Autodesk Inventor part; units mm, degrees
(part 2 of 4)
  line L810 (39.2782, -35.709) -> (37.2782, -35.709)
  line L811 (36.2782, -33.9769) -> (37.2782, -32.2449)
  line L812 (42.0103, -32.9769) -> (41.0103, -31.2449)
  line L813 (44.0103, -32.9769) -> (42.0103, -32.9769)
  line L814 (45.0103, -31.2449) -> (44.0103, -32.9769)
  line L815 (41.0103, -31.2449) -> (42.0103, -29.5128)
  line L816 (42.0103, -29.5128) -> (44.0103, -29.5128)
  line L817 (44.0103, -29.5128) -> (45.0103, -31.2449)
  line L818 (46.7423, -35.709) -> (45.7423, -33.9769)
  line L819 (49.7423, -33.9769) -> (48.7423, -35.709)
  line L820 (46.7423, -32.2449) -> (48.7423, -32.2449)
  line L821 (48.7423, -32.2449) -> (49.7423, -33.9769)
  line L822 (48.7423, -35.709) -> (46.7423, -35.709)
  line L823 (45.7423, -33.9769) -> (46.7423, -32.2449)
  line L824 (51.4744, -32.9769) -> (50.4744, -31.2449)
  line L825 (53.4744, -32.9769) -> (51.4744, -32.9769)
  line L826 (54.4744, -31.2449) -> (53.4744, -32.9769)
  line L827 (50.4744, -31.2449) -> (51.4744, -29.5128)
  line L828 (51.4744, -29.5128) -> (53.4744, -29.5128)
  line L829 (53.4744, -29.5128) -> (54.4744, -31.2449)
  line L830 (56.2064, -35.709) -> (55.2064, -33.9769)
  line L831 (59.2064, -33.9769) -> (58.2064, -35.709)
  line L832 (56.2064, -32.2449) -> (58.2064, -32.2449)
  line L833 (58.2064, -32.2449) -> (59.2064, -33.9769)
  line L834 (58.2064, -35.709) -> (56.2064, -35.709)
  line L835 (55.2064, -33.9769) -> (56.2064, -32.2449)
  line L836 (60.9385, -32.9769) -> (59.9385, -31.2449)
  line L837 (62.9385, -32.9769) -> (60.9385, -32.9769)
  line L838 (63.9385, -31.2449) -> (62.9385, -32.9769)
  line L839 (59.9385, -31.2449) -> (60.9385, -29.5128)
  line L840 (60.9385, -29.5128) -> (62.9385, -29.5128)
  line L841 (62.9385, -29.5128) -> (63.9385, -31.2449)
  line L842 (65.6705, -35.709) -> (64.6705, -33.9769)
  line L843 (68.6705, -33.9769) -> (67.6705, -35.709)
  line L844 (65.6705, -32.2449) -> (67.6705, -32.2449)
  line L845 (67.6705, -32.2449) -> (68.6705, -33.9769)
  line L846 (67.6705, -35.709) -> (65.6705, -35.709)
  line L847 (64.6705, -33.9769) -> (65.6705, -32.2449)
  line L848 (70.4026, -32.9769) -> (69.4026, -31.2449)
  line L849 (72.4026, -32.9769) -> (70.4026, -32.9769)
  line L850 (73.4026, -31.2449) -> (72.4026, -32.9769)
  line L851 (69.4026, -31.2449) -> (70.4026, -29.5128)
  line L852 (70.4026, -29.5128) -> (72.4026, -29.5128)
  line L853 (72.4026, -29.5128) -> (73.4026, -31.2449)
  line L854 (75.1346, -35.709) -> (74.1346, -33.9769)
  line L855 (78.1346, -33.9769) -> (77.1346, -35.709)
  line L856 (75.1346, -32.2449) -> (77.1346, -32.2449)
  line L857 (77.1346, -32.2449) -> (78.1346, -33.9769)
  line L858 (77.1346, -35.709) -> (75.1346, -35.709)
  line L859 (74.1346, -33.9769) -> (75.1346, -32.2449)
  line L860 (79.8667, -32.9769) -> (78.8667, -31.2449)
  line L861 (81.8667, -32.9769) -> (79.8667, -32.9769)
  line L862 (82.8667, -31.2449) -> (81.8667, -32.9769)
  line L863 (78.8667, -31.2449) -> (79.8667, -29.5128)
  line L864 (79.8667, -29.5128) -> (81.8667, -29.5128)
  line L865 (81.8667, -29.5128) -> (82.8667, -31.2449)
  line L866 (18.35, -41.1731) -> (17.35, -39.441)
  line L867 (21.35, -39.441) -> (20.35, -41.1731)
  line L868 (18.35, -37.709) -> (20.35, -37.709)
  line L869 (20.35, -37.709) -> (21.35, -39.441)
  line L870 (20.35, -41.1731) -> (18.35, -41.1731)
  line L871 (17.35, -39.441) -> (18.35, -37.709)
  line L872 (23.0821, -38.441) -> (22.0821, -36.709)
  line L873 (25.0821, -38.441) -> (23.0821, -38.441)
  line L874 (26.0821, -36.709) -> (25.0821, -38.441)
  line L875 (22.0821, -36.709) -> (23.0821, -34.9769)
  line L876 (23.0821, -34.9769) -> (25.0821, -34.9769)
  line L877 (25.0821, -34.9769) -> (26.0821, -36.709)
  line L878 (27.8141, -41.1731) -> (26.8141, -39.441)
  line L879 (30.8141, -39.441) -> (29.8141, -41.1731)
  line L880 (27.8141, -37.709) -> (29.8141, -37.709)
  line L881 (29.8141, -37.709) -> (30.8141, -39.441)
  line L882 (29.8141, -41.1731) -> (27.8141, -41.1731)
  line L883 (26.8141, -39.441) -> (27.8141, -37.709)
  line L884 (32.5462, -38.441) -> (31.5462, -36.709)
  line L885 (34.5462, -38.441) -> (32.5462, -38.441)
  line L886 (35.5462, -36.709) -> (34.5462, -38.441)
  line L887 (31.5462, -36.709) -> (32.5462, -34.9769)
  line L888 (32.5462, -34.9769) -> (34.5462, -34.9769)
  line L889 (34.5462, -34.9769) -> (35.5462, -36.709)
  line L890 (37.2782, -41.1731) -> (36.2782, -39.441)
  line L891 (40.2782, -39.441) -> (39.2782, -41.1731)
  line L892 (37.2782, -37.709) -> (39.2782, -37.709)
  line L893 (39.2782, -37.709) -> (40.2782, -39.441)
  line L894 (39.2782, -41.1731) -> (37.2782, -41.1731)
  line L895 (36.2782, -39.441) -> (37.2782, -37.709)
  line L896 (42.0103, -38.441) -> (41.0103, -36.709)
  line L897 (44.0103, -38.441) -> (42.0103, -38.441)
  line L898 (45.0103, -36.709) -> (44.0103, -38.441)
  line L899 (41.0103, -36.709) -> (42.0103, -34.9769)
  line L900 (42.0103, -34.9769) -> (44.0103, -34.9769)
  line L901 (44.0103, -34.9769) -> (45.0103, -36.709)
  line L902 (46.7423, -41.1731) -> (45.7423, -39.441)
  line L903 (49.7423, -39.441) -> (48.7423, -41.1731)
  line L904 (46.7423, -37.709) -> (48.7423, -37.709)
  line L905 (48.7423, -37.709) -> (49.7423, -39.441)
  line L906 (48.7423, -41.1731) -> (46.7423, -41.1731)
  line L907 (45.7423, -39.441) -> (46.7423, -37.709)
  line L908 (51.4744, -38.441) -> (50.4744, -36.709)
  line L909 (53.4744, -38.441) -> (51.4744, -38.441)
  line L910 (54.4744, -36.709) -> (53.4744, -38.441)
  line L911 (50.4744, -36.709) -> (51.4744, -34.9769)
  line L912 (51.4744, -34.9769) -> (53.4744, -34.9769)
  line L913 (53.4744, -34.9769) -> (54.4744, -36.709)
  line L914 (56.2064, -41.1731) -> (55.2064, -39.441)
  line L915 (59.2064, -39.441) -> (58.2064, -41.1731)
  line L916 (56.2064, -37.709) -> (58.2064, -37.709)
  line L917 (58.2064, -37.709) -> (59.2064, -39.441)
  line L918 (58.2064, -41.1731) -> (56.2064, -41.1731)
  line L919 (55.2064, -39.441) -> (56.2064, -37.709)
  line L920 (60.9385, -38.441) -> (59.9385, -36.709)
  line L921 (62.9385, -38.441) -> (60.9385, -38.441)
  line L922 (63.9385, -36.709) -> (62.9385, -38.441)
  line L923 (59.9385, -36.709) -> (60.9385, -34.9769)
  line L924 (60.9385, -34.9769) -> (62.9385, -34.9769)
  line L925 (62.9385, -34.9769) -> (63.9385, -36.709)
  line L926 (65.6705, -41.1731) -> (64.6705, -39.441)
  line L927 (68.6705, -39.441) -> (67.6705, -41.1731)
  line L928 (65.6705, -37.709) -> (67.6705, -37.709)
  line L929 (67.6705, -37.709) -> (68.6705, -39.441)
  line L930 (67.6705, -41.1731) -> (65.6705, -41.1731)
  line L931 (64.6705, -39.441) -> (65.6705, -37.709)
  line L932 (70.4026, -38.441) -> (69.4026, -36.709)
  line L933 (72.4026, -38.441) -> (70.4026, -38.441)
  line L934 (73.4026, -36.709) -> (72.4026, -38.441)
  line L935 (69.4026, -36.709) -> (70.4026, -34.9769)
  line L936 (70.4026, -34.9769) -> (72.4026, -34.9769)
  line L937 (72.4026, -34.9769) -> (73.4026, -36.709)
  line L938 (75.1346, -41.1731) -> (74.1346, -39.441)
  line L939 (78.1346, -39.441) -> (77.1346, -41.1731)
  line L940 (75.1346, -37.709) -> (77.1346, -37.709)
  line L941 (77.1346, -37.709) -> (78.1346, -39.441)
  line L942 (77.1346, -41.1731) -> (75.1346, -41.1731)
  line L943 (74.1346, -39.441) -> (75.1346, -37.709)
  line L944 (79.8667, -38.441) -> (78.8667, -36.709)
  line L945 (81.8667, -38.441) -> (79.8667, -38.441)
  line L946 (82.8667, -36.709) -> (81.8667, -38.441)
  line L947 (78.8667, -36.709) -> (79.8667, -34.9769)
  line L948 (79.8667, -34.9769) -> (81.8667, -34.9769)
  line L949 (81.8667, -34.9769) -> (82.8667, -36.709)
  line L950 (18.35, -46.6372) -> (17.35, -44.9051)
  line L951 (21.35, -44.9051) -> (20.35, -46.6372)
  line L952 (18.35, -43.1731) -> (20.35, -43.1731)
  line L953 (20.35, -43.1731) -> (21.35, -44.9051)
  line L954 (20.35, -46.6372) -> (18.35, -46.6372)
  line L955 (17.35, -44.9051) -> (18.35, -43.1731)
  line L956 (23.0821, -43.9051) -> (22.0821, -42.1731)
  line L957 (25.0821, -43.9051) -> (23.0821, -43.9051)
  line L958 (26.0821, -42.1731) -> (25.0821, -43.9051)
  line L959 (22.0821, -42.1731) -> (23.0821, -40.441)
  line L960 (23.0821, -40.441) -> (25.0821, -40.441)
  line L961 (25.0821, -40.441) -> (26.0821, -42.1731)
  line L962 (27.8141, -46.6372) -> (26.8141, -44.9051)
  line L963 (30.8141, -44.9051) -> (29.8141, -46.6372)
  line L964 (27.8141, -43.1731) -> (29.8141, -43.1731)
  line L965 (29.8141, -43.1731) -> (30.8141, -44.9051)
  line L966 (29.8141, -46.6372) -> (27.8141, -46.6372)
  line L967 (26.8141, -44.9051) -> (27.8141, -43.1731)
  line L968 (32.5462, -43.9051) -> (31.5462, -42.1731)
  line L969 (34.5462, -43.9051) -> (32.5462, -43.9051)
  line L970 (35.5462, -42.1731) -> (34.5462, -43.9051)
  line L971 (31.5462, -42.1731) -> (32.5462, -40.441)
  line L972 (32.5462, -40.441) -> (34.5462, -40.441)
  line L973 (34.5462, -40.441) -> (35.5462, -42.1731)
  line L974 (37.2782, -46.6372) -> (36.2782, -44.9051)
  line L975 (40.2782, -44.9051) -> (39.2782, -46.6372)
  line L976 (37.2782, -43.1731) -> (39.2782, -43.1731)
  line L977 (39.2782, -43.1731) -> (40.2782, -44.9051)
  line L978 (39.2782, -46.6372) -> (37.2782, -46.6372)
  line L979 (36.2782, -44.9051) -> (37.2782, -43.1731)
  line L980 (42.0103, -43.9051) -> (41.0103, -42.1731)
  line L981 (44.0103, -43.9051) -> (42.0103, -43.9051)
  line L982 (45.0103, -42.1731) -> (44.0103, -43.9051)
  line L983 (41.0103, -42.1731) -> (42.0103, -40.441)
  line L984 (42.0103, -40.441) -> (44.0103, -40.441)
  line L985 (44.0103, -40.441) -> (45.0103, -42.1731)
  line L986 (46.7423, -46.6372) -> (45.7423, -44.9051)
  line L987 (49.7423, -44.9051) -> (48.7423, -46.6372)
  line L988 (46.7423, -43.1731) -> (48.7423, -43.1731)
  line L989 (48.7423, -43.1731) -> (49.7423, -44.9051)
  line L990 (48.7423, -46.6372) -> (46.7423, -46.6372)
  line L991 (45.7423, -44.9051) -> (46.7423, -43.1731)
  line L992 (51.4744, -43.9051) -> (50.4744, -42.1731)
  line L993 (53.4744, -43.9051) -> (51.4744, -43.9051)
  line L994 (54.4744, -42.1731) -> (53.4744, -43.9051)
  line L995 (50.4744, -42.1731) -> (51.4744, -40.441)
  line L996 (51.4744, -40.441) -> (53.4744, -40.441)
  line L997 (53.4744, -40.441) -> (54.4744, -42.1731)
  line L998 (56.2064, -46.6372) -> (55.2064, -44.9051)
  line L999 (59.2064, -44.9051) -> (58.2064, -46.6372)
  line L1000 (56.2064, -43.1731) -> (58.2064, -43.1731)
  line L1001 (58.2064, -43.1731) -> (59.2064, -44.9051)
  line L1002 (58.2064, -46.6372) -> (56.2064, -46.6372)
  line L1003 (55.2064, -44.9051) -> (56.2064, -43.1731)
  line L1004 (60.9385, -43.9051) -> (59.9385, -42.1731)
  line L1005 (62.9385, -43.9051) -> (60.9385, -43.9051)
  line L1006 (63.9385, -42.1731) -> (62.9385, -43.9051)
  line L1007 (59.9385, -42.1731) -> (60.9385, -40.441)
  line L1008 (60.9385, -40.441) -> (62.9385, -40.441)
  line L1009 (62.9385, -40.441) -> (63.9385, -42.1731)
  line L1010 (65.6705, -46.6372) -> (64.6705, -44.9051)
  line L1011 (68.6705, -44.9051) -> (67.6705, -46.6372)
  line L1012 (65.6705, -43.1731) -> (67.6705, -43.1731)
  line L1013 (67.6705, -43.1731) -> (68.6705, -44.9051)
  line L1014 (67.6705, -46.6372) -> (65.6705, -46.6372)
  line L1015 (64.6705, -44.9051) -> (65.6705, -43.1731)
  line L1016 (70.4026, -43.9051) -> (69.4026, -42.1731)
  line L1017 (72.4026, -43.9051) -> (70.4026, -43.9051)
  line L1018 (73.4026, -42.1731) -> (72.4026, -43.9051)
  line L1019 (69.4026, -42.1731) -> (70.4026, -40.441)
  line L1020 (70.4026, -40.441) -> (72.4026, -40.441)
  line L1021 (72.4026, -40.441) -> (73.4026, -42.1731)
  line L1022 (75.1346, -46.6372) -> (74.1346, -44.9051)
  line L1023 (78.1346, -44.9051) -> (77.1346, -46.6372)
  line L1024 (75.1346, -43.1731) -> (77.1346, -43.1731)
  line L1025 (77.1346, -43.1731) -> (78.1346, -44.9051)
  line L1026 (77.1346, -46.6372) -> (75.1346, -46.6372)
  line L1027 (74.1346, -44.9051) -> (75.1346, -43.1731)
  line L1028 (79.8667, -43.9051) -> (78.8667, -42.1731)
  line L1029 (81.8667, -43.9051) -> (79.8667, -43.9051)
  line L1030 (82.8667, -42.1731) -> (81.8667, -43.9051)
  line L1031 (78.8667, -42.1731) -> (79.8667, -40.441)
  line L1032 (79.8667, -40.441) -> (81.8667, -40.441)
  line L1033 (81.8667, -40.441) -> (82.8667, -42.1731)
  line L1034 (18.35, -52.1013) -> (17.35, -50.3692)
  line L1035 (21.35, -50.3692) -> (20.35, -52.1013)
  line L1036 (18.35, -48.6372) -> (20.35, -48.6372)
  line L1037 (20.35, -48.6372) -> (21.35, -50.3692)
  line L1038 (20.35, -52.1013) -> (18.35, -52.1013)
  line L1039 (17.35, -50.3692) -> (18.35, -48.6372)
  line L1040 (23.0821, -49.3692) -> (22.0821, -47.6372)
  line L1041 (25.0821, -49.3692) -> (23.0821, -49.3692)
  line L1042 (26.0821, -47.6372) -> (25.0821, -49.3692)
  line L1043 (22.0821, -47.6372) -> (23.0821, -45.9051)
  line L1044 (23.0821, -45.9051) -> (25.0821, -45.9051)
  line L1045 (25.0821, -45.9051) -> (26.0821, -47.6372)
  line L1046 (27.8141, -52.1013) -> (26.8141, -50.3692)
  line L1047 (30.8141, -50.3692) -> (29.8141, -52.1013)
  line L1048 (27.8141, -48.6372) -> (29.8141, -48.6372)
  line L1049 (29.8141, -48.6372) -> (30.8141, -50.3692)
  line L1050 (29.8141, -52.1013) -> (27.8141, -52.1013)
  line L1051 (26.8141, -50.3692) -> (27.8141, -48.6372)
  line L1052 (32.5462, -49.3692) -> (31.5462, -47.6372)
  line L1053 (34.5462, -49.3692) -> (32.5462, -49.3692)
  line L1054 (35.5462, -47.6372) -> (34.5462, -49.3692)
  line L1055 (31.5462, -47.6372) -> (32.5462, -45.9051)
  line L1056 (32.5462, -45.9051) -> (34.5462, -45.9051)
  line L1057 (34.5462, -45.9051) -> (35.5462, -47.6372)
  line L1058 (37.2782, -52.1013) -> (36.2782, -50.3692)
  line L1059 (40.2782, -50.3692) -> (39.2782, -52.1013)
  line L1060 (37.2782, -48.6372) -> (39.2782, -48.6372)
  line L1061 (39.2782, -48.6372) -> (40.2782, -50.3692)
  line L1062 (39.2782, -52.1013) -> (37.2782, -52.1013)
  line L1063 (36.2782, -50.3692) -> (37.2782, -48.6372)
  line L1064 (42.0103, -49.3692) -> (41.0103, -47.6372)
  line L1065 (44.0103, -49.3692) -> (42.0103, -49.3692)
  line L1066 (45.0103, -47.6372) -> (44.0103, -49.3692)
  line L1067 (41.0103, -47.6372) -> (42.0103, -45.9051)
  line L1068 (42.0103, -45.9051) -> (44.0103, -45.9051)
  line L1069 (44.0103, -45.9051) -> (45.0103, -47.6372)
  line L1070 (46.7423, -52.1013) -> (45.7423, -50.3692)
  line L1071 (49.7423, -50.3692) -> (48.7423, -52.1013)
  line L1072 (46.7423, -48.6372) -> (48.7423, -48.6372)
  line L1073 (48.7423, -48.6372) -> (49.7423, -50.3692)
  line L1074 (48.7423, -52.1013) -> (46.7423, -52.1013)
  line L1075 (45.7423, -50.3692) -> (46.7423, -48.6372)
  line L1076 (51.4744, -49.3692) -> (50.4744, -47.6372)
  line L1077 (53.4744, -49.3692) -> (51.4744, -49.3692)
  line L1078 (54.4744, -47.6372) -> (53.4744, -49.3692)
  line L1079 (50.4744, -47.6372) -> (51.4744, -45.9051)
  line L1080 (51.4744, -45.9051) -> (53.4744, -45.9051)
  line L1081 (53.4744, -45.9051) -> (54.4744, -47.6372)
  line L1082 (56.2064, -52.1013) -> (55.2064, -50.3692)
  line L1083 (59.2064, -50.3692) -> (58.2064, -52.1013)
  line L1084 (56.2064, -48.6372) -> (58.2064, -48.6372)
  line L1085 (58.2064, -48.6372) -> (59.2064, -50.3692)
  line L1086 (58.2064, -52.1013) -> (56.2064, -52.1013)
  line L1087 (55.2064, -50.3692) -> (56.2064, -48.6372)
  line L1088 (60.9385, -49.3692) -> (59.9385, -47.6372)
  line L1089 (62.9385, -49.3692) -> (60.9385, -49.3692)
  line L1090 (63.9385, -47.6372) -> (62.9385, -49.3692)
  line L1091 (59.9385, -47.6372) -> (60.9385, -45.9051)
  line L1092 (60.9385, -45.9051) -> (62.9385, -45.9051)
  line L1093 (62.9385, -45.9051) -> (63.9385, -47.6372)
  line L1094 (65.6705, -52.1013) -> (64.6705, -50.3692)
  line L1095 (68.6705, -50.3692) -> (67.6705, -52.1013)
  line L1096 (65.6705, -48.6372) -> (67.6705, -48.6372)
  line L1097 (67.6705, -48.6372) -> (68.6705, -50.3692)
  line L1098 (67.6705, -52.1013) -> (65.6705, -52.1013)
  line L1099 (64.6705, -50.3692) -> (65.6705, -48.6372)
  line L1100 (70.4026, -49.3692) -> (69.4026, -47.6372)
  line L1101 (72.4026, -49.3692) -> (70.4026, -49.3692)
  line L1102 (73.4026, -47.6372) -> (72.4026, -49.3692)
  line L1103 (69.4026, -47.6372) -> (70.4026, -45.9051)
  line L1104 (70.4026, -45.9051) -> (72.4026, -45.9051)
  line L1105 (72.4026, -45.9051) -> (73.4026, -47.6372)
  line L1106 (75.1346, -52.1013) -> (74.1346, -50.3692)
  line L1107 (78.1346, -50.3692) -> (77.1346, -52.1013)
  line L1108 (75.1346, -48.6372) -> (77.1346, -48.6372)
  line L1109 (77.1346, -48.6372) -> (78.1346, -50.3692)
  line L1110 (77.1346, -52.1013) -> (75.1346, -52.1013)
  line L1111 (74.1346, -50.3692) -> (75.1346, -48.6372)
  line L1112 (79.8667, -49.3692) -> (78.8667, -47.6372)
  line L1113 (81.8667, -49.3692) -> (79.8667, -49.3692)
  line L1114 (82.8667, -47.6372) -> (81.8667, -49.3692)
  line L1115 (78.8667, -47.6372) -> (79.8667, -45.9051)
  line L1116 (79.8667, -45.9051) -> (81.8667, -45.9051)
  line L1117 (81.8667, -45.9051) -> (82.8667, -47.6372)
  line L1118 (18.35, -57.5654) -> (17.35, -55.8333)
  line L1119 (21.35, -55.8333) -> (20.35, -57.5654)
  line L1120 (18.35, -54.1013) -> (20.35, -54.1013)
  line L1121 (20.35, -54.1013) -> (21.35, -55.8333)
  line L1122 (20.35, -57.5654) -> (18.35, -57.5654)
  line L1123 (17.35, -55.8333) -> (18.35, -54.1013)
  line L1124 (23.0821, -54.8333) -> (22.0821, -53.1013)
  line L1125 (25.0821, -54.8333) -> (23.0821, -54.8333)
  line L1126 (26.0821, -53.1013) -> (25.0821, -54.8333)
  line L1127 (22.0821, -53.1013) -> (23.0821, -51.3692)
  line L1128 (23.0821, -51.3692) -> (25.0821, -51.3692)
  line L1129 (25.0821, -51.3692) -> (26.0821, -53.1013)
  line L1130 (27.8141, -57.5654) -> (26.8141, -55.8333)
  line L1131 (30.8141, -55.8333) -> (29.8141, -57.5654)
  line L1132 (27.8141, -54.1013) -> (29.8141, -54.1013)
  line L1133 (29.8141, -54.1013) -> (30.8141, -55.8333)
  line L1134 (29.8141, -57.5654) -> (27.8141, -57.5654)
  line L1135 (26.8141, -55.8333) -> (27.8141, -54.1013)
  line L1136 (32.5462, -54.8333) -> (31.5462, -53.1013)
  line L1137 (34.5462, -54.8333) -> (32.5462, -54.8333)
  line L1138 (35.5462, -53.1013) -> (34.5462, -54.8333)
  line L1139 (31.5462, -53.1013) -> (32.5462, -51.3692)
  line L1140 (32.5462, -51.3692) -> (34.5462, -51.3692)
  line L1141 (34.5462, -51.3692) -> (35.5462, -53.1013)
  line L1142 (37.2782, -57.5654) -> (36.2782, -55.8333)
  line L1143 (40.2782, -55.8333) -> (39.2782, -57.5654)
  line L1144 (37.2782, -54.1013) -> (39.2782, -54.1013)
  line L1145 (39.2782, -54.1013) -> (40.2782, -55.8333)
  line L1146 (39.2782, -57.5654) -> (37.2782, -57.5654)
  line L1147 (36.2782, -55.8333) -> (37.2782, -54.1013)
  line L1148 (42.0103, -54.8333) -> (41.0103, -53.1013)
  line L1149 (44.0103, -54.8333) -> (42.0103, -54.8333)
  line L1150 (45.0103, -53.1013) -> (44.0103, -54.8333)
  line L1151 (41.0103, -53.1013) -> (42.0103, -51.3692)
  line L1152 (42.0103, -51.3692) -> (44.0103, -51.3692)
  line L1153 (44.0103, -51.3692) -> (45.0103, -53.1013)
  line L1154 (46.7423, -57.5654) -> (45.7423, -55.8333)
  line L1155 (49.7423, -55.8333) -> (48.7423, -57.5654)
  line L1156 (46.7423, -54.1013) -> (48.7423, -54.1013)
  line L1157 (48.7423, -54.1013) -> (49.7423, -55.8333)
  line L1158 (48.7423, -57.5654) -> (46.7423, -57.5654)
  line L1159 (45.7423, -55.8333) -> (46.7423, -54.1013)
  line L1160 (51.4744, -54.8333) -> (50.4744, -53.1013)
  line L1161 (53.4744, -54.8333) -> (51.4744, -54.8333)
  line L1162 (54.4744, -53.1013) -> (53.4744, -54.8333)
  line L1163 (50.4744, -53.1013) -> (51.4744, -51.3692)
  line L1164 (51.4744, -51.3692) -> (53.4744, -51.3692)
  line L1165 (53.4744, -51.3692) -> (54.4744, -53.1013)
  line L1166 (56.2064, -57.5654) -> (55.2064, -55.8333)
  line L1167 (59.2064, -55.8333) -> (58.2064, -57.5654)
  line L1168 (56.2064, -54.1013) -> (58.2064, -54.1013)
  line L1169 (58.2064, -54.1013) -> (59.2064, -55.8333)
  line L1170 (58.2064, -57.5654) -> (56.2064, -57.5654)
  line L1171 (55.2064, -55.8333) -> (56.2064, -54.1013)
  line L1172 (60.9385, -54.8333) -> (59.9385, -53.1013)
  line L1173 (62.9385, -54.8333) -> (60.9385, -54.8333)
  line L1174 (63.9385, -53.1013) -> (62.9385, -54.8333)
  line L1175 (59.9385, -53.1013) -> (60.9385, -51.3692)
  line L1176 (60.9385, -51.3692) -> (62.9385, -51.3692)
  line L1177 (62.9385, -51.3692) -> (63.9385, -53.1013)
  line L1178 (65.6705, -57.5654) -> (64.6705, -55.8333)
  line L1179 (68.6705, -55.8333) -> (67.6705, -57.5654)
  line L1180 (65.6705, -54.1013) -> (67.6705, -54.1013)
  line L1181 (67.6705, -54.1013) -> (68.6705, -55.8333)
  line L1182 (67.6705, -57.5654) -> (65.6705, -57.5654)
  line L1183 (64.6705, -55.8333) -> (65.6705, -54.1013)
  line L1184 (70.4026, -54.8333) -> (69.4026, -53.1013)
  line L1185 (72.4026, -54.8333) -> (70.4026, -54.8333)
  line L1186 (73.4026, -53.1013) -> (72.4026, -54.8333)
  line L1187 (69.4026, -53.1013) -> (70.4026, -51.3692)
  line L1188 (70.4026, -51.3692) -> (72.4026, -51.3692)
  line L1189 (72.4026, -51.3692) -> (73.4026, -53.1013)
  line L1190 (75.1346, -57.5654) -> (74.1346, -55.8333)
  line L1191 (78.1346, -55.8333) -> (77.1346, -57.5654)
  line L1192 (75.1346, -54.1013) -> (77.1346, -54.1013)
  line L1193 (77.1346, -54.1013) -> (78.1346, -55.8333)
  line L1194 (77.1346, -57.5654) -> (75.1346, -57.5654)
  line L1195 (74.1346, -55.8333) -> (75.1346, -54.1013)
  line L1196 (79.8667, -54.8333) -> (78.8667, -53.1013)
  line L1197 (81.8667, -54.8333) -> (79.8667, -54.8333)
  line L1198 (82.8667, -53.1013) -> (81.8667, -54.8333)
  line L1199 (78.8667, -53.1013) -> (79.8667, -51.3692)
  line L1200 (79.8667, -51.3692) -> (81.8667, -51.3692)
  line L1201 (81.8667, -51.3692) -> (82.8667, -53.1013)
  line L1202 (18.35, -63.0295) -> (17.35, -61.2974)
  line L1203 (21.35, -61.2974) -> (20.35, -63.0295)
  line L1204 (18.35, -59.5654) -> (20.35, -59.5654)
  line L1205 (20.35, -59.5654) -> (21.35, -61.2974)
  line L1206 (20.35, -63.0295) -> (18.35, -63.0295)
  line L1207 (17.35, -61.2974) -> (18.35, -59.5654)
  line L1208 (23.0821, -60.2974) -> (22.0821, -58.5654)
  line L1209 (25.0821, -60.2974) -> (23.0821, -60.2974)
  line L1210 (26.0821, -58.5654) -> (25.0821, -60.2974)
  line L1211 (22.0821, -58.5654) -> (23.0821, -56.8333)
  line L1212 (23.0821, -56.8333) -> (25.0821, -56.8333)
  line L1213 (25.0821, -56.8333) -> (26.0821, -58.5654)
  line L1214 (27.8141, -63.0295) -> (26.8141, -61.2974)
  line L1215 (30.8141, -61.2974) -> (29.8141, -63.0295)
  line L1216 (27.8141, -59.5654) -> (29.8141, -59.5654)
  line L1217 (29.8141, -59.5654) -> (30.8141, -61.2974)
  line L1218 (29.8141, -63.0295) -> (27.8141, -63.0295)
  line L1219 (26.8141, -61.2974) -> (27.8141, -59.5654)
  line L1220 (32.5462, -60.2974) -> (31.5462, -58.5654)
  line L1221 (34.5462, -60.2974) -> (32.5462, -60.2974)
  line L1222 (35.5462, -58.5654) -> (34.5462, -60.2974)
  line L1223 (31.5462, -58.5654) -> (32.5462, -56.8333)
  line L1224 (32.5462, -56.8333) -> (34.5462, -56.8333)
  line L1225 (34.5462, -56.8333) -> (35.5462, -58.5654)
  line L1226 (37.2782, -63.0295) -> (36.2782, -61.2974)
  line L1227 (40.2782, -61.2974) -> (39.2782, -63.0295)
  line L1228 (37.2782, -59.5654) -> (39.2782, -59.5654)
  line L1229 (39.2782, -59.5654) -> (40.2782, -61.2974)
  line L1230 (39.2782, -63.0295) -> (37.2782, -63.0295)
  line L1231 (36.2782, -61.2974) -> (37.2782, -59.5654)
  line L1232 (42.0103, -60.2974) -> (41.0103, -58.5654)
  line L1233 (44.0103, -60.2974) -> (42.0103, -60.2974)
  line L1234 (45.0103, -58.5654) -> (44.0103, -60.2974)
  line L1235 (41.0103, -58.5654) -> (42.0103, -56.8333)
  line L1236 (42.0103, -56.8333) -> (44.0103, -56.8333)
  line L1237 (44.0103, -56.8333) -> (45.0103, -58.5654)
  line L1238 (46.7423, -63.0295) -> (45.7423, -61.2974)
  line L1239 (49.7423, -61.2974) -> (48.7423, -63.0295)
  line L1240 (46.7423, -59.5654) -> (48.7423, -59.5654)
  line L1241 (48.7423, -59.5654) -> (49.7423, -61.2974)
  line L1242 (48.7423, -63.0295) -> (46.7423, -63.0295)
  line L1243 (45.7423, -61.2974) -> (46.7423, -59.5654)
  line L1244 (51.4744, -60.2974) -> (50.4744, -58.5654)
  line L1245 (53.4744, -60.2974) -> (51.4744, -60.2974)
  line L1246 (54.4744, -58.5654) -> (53.4744, -60.2974)
  line L1247 (50.4744, -58.5654) -> (51.4744, -56.8333)
  line L1248 (51.4744, -56.8333) -> (53.4744, -56.8333)
  line L1249 (53.4744, -56.8333) -> (54.4744, -58.5654)
  line L1250 (56.2064, -63.0295) -> (55.2064, -61.2974)
  line L1251 (59.2064, -61.2974) -> (58.2064, -63.0295)
  line L1252 (56.2064, -59.5654) -> (58.2064, -59.5654)
  line L1253 (58.2064, -59.5654) -> (59.2064, -61.2974)
  line L1254 (58.2064, -63.0295) -> (56.2064, -63.0295)
  line L1255 (55.2064, -61.2974) -> (56.2064, -59.5654)
  line L1256 (60.9385, -60.2974) -> (59.9385, -58.5654)
  line L1257 (62.9385, -60.2974) -> (60.9385, -60.2974)
  line L1258 (63.9385, -58.5654) -> (62.9385, -60.2974)
  line L1259 (59.9385, -58.5654) -> (60.9385, -56.8333)
  line L1260 (60.9385, -56.8333) -> (62.9385, -56.8333)
  line L1261 (62.9385, -56.8333) -> (63.9385, -58.5654)
  line L1262 (65.6705, -63.0295) -> (64.6705, -61.2974)
  line L1263 (68.6705, -61.2974) -> (67.6705, -63.0295)
  line L1264 (65.6705, -59.5654) -> (67.6705, -59.5654)
  line L1265 (67.6705, -59.5654) -> (68.6705, -61.2974)
  line L1266 (67.6705, -63.0295) -> (65.6705, -63.0295)
  line L1267 (64.6705, -61.2974) -> (65.6705, -59.5654)
  line L1268 (70.4026, -60.2974) -> (69.4026, -58.5654)
  line L1269 (72.4026, -60.2974) -> (70.4026, -60.2974)
  line L1270 (73.4026, -58.5654) -> (72.4026, -60.2974)
  line L1271 (69.4026, -58.5654) -> (70.4026, -56.8333)
  line L1272 (70.4026, -56.8333) -> (72.4026, -56.8333)
  line L1273 (72.4026, -56.8333) -> (73.4026, -58.5654)
  line L1274 (75.1346, -63.0295) -> (74.1346, -61.2974)
  line L1275 (78.1346, -61.2974) -> (77.1346, -63.0295)
  line L1276 (75.1346, -59.5654) -> (77.1346, -59.5654)
  line L1277 (77.1346, -59.5654) -> (78.1346, -61.2974)
  line L1278 (77.1346, -63.0295) -> (75.1346, -63.0295)
  line L1279 (74.1346, -61.2974) -> (75.1346, -59.5654)
  line L1280 (79.8667, -60.2974) -> (78.8667, -58.5654)
  line L1281 (81.8667, -60.2974) -> (79.8667, -60.2974)
  line L1282 (82.8667, -58.5654) -> (81.8667, -60.2974)
  line L1283 (78.8667, -58.5654) -> (79.8667, -56.8333)
  line L1284 (79.8667, -56.8333) -> (81.8667, -56.8333)
  line L1285 (81.8667, -56.8333) -> (82.8667, -58.5654)
  line L1286 (18.35, -68.4936) -> (17.35, -66.7615)
  line L1287 (21.35, -66.7615) -> (20.35, -68.4936)
  line L1288 (18.35, -65.0295) -> (20.35, -65.0295)
  line L1289 (20.35, -65.0295) -> (21.35, -66.7615)
  line L1290 (20.35, -68.4936) -> (18.35, -68.4936)
  line L1291 (17.35, -66.7615) -> (18.35, -65.0295)
  line L1292 (23.0821, -65.7615) -> (22.0821, -64.0295)
  line L1293 (25.0821, -65.7615) -> (23.0821, -65.7615)
  line L1294 (26.0821, -64.0295) -> (25.0821, -65.7615)
  line L1295 (22.0821, -64.0295) -> (23.0821, -62.2974)
  line L1296 (23.0821, -62.2974) -> (25.0821, -62.2974)
  line L1297 (25.0821, -62.2974) -> (26.0821, -64.0295)
  line L1298 (27.8141, -68.4936) -> (26.8141, -66.7615)
  line L1299 (30.8141, -66.7615) -> (29.8141, -68.4936)
  line L1300 (27.8141, -65.0295) -> (29.8141, -65.0295)
  line L1301 (29.8141, -65.0295) -> (30.8141, -66.7615)
  line L1302 (29.8141, -68.4936) -> (27.8141, -68.4936)
  line L1303 (26.8141, -66.7615) -> (27.8141, -65.0295)
  line L1304 (32.5462, -65.7615) -> (31.5462, -64.0295)
  line L1305 (34.5462, -65.7615) -> (32.5462, -65.7615)
  line L1306 (35.5462, -64.0295) -> (34.5462, -65.7615)
  line L1307 (31.5462, -64.0295) -> (32.5462, -62.2974)
  line L1308 (32.5462, -62.2974) -> (34.5462, -62.2974)
  line L1309 (34.5462, -62.2974) -> (35.5462, -64.0295)
  line L1310 (37.2782, -68.4936) -> (36.2782, -66.7615)
  line L1311 (40.2782, -66.7615) -> (39.2782, -68.4936)
  line L1312 (37.2782, -65.0295) -> (39.2782, -65.0295)
  line L1313 (39.2782, -65.0295) -> (40.2782, -66.7615)
  line L1314 (39.2782, -68.4936) -> (37.2782, -68.4936)
  line L1315 (36.2782, -66.7615) -> (37.2782, -65.0295)
  line L1316 (42.0103, -65.7615) -> (41.0103, -64.0295)
  line L1317 (44.0103, -65.7615) -> (42.0103, -65.7615)
  line L1318 (45.0103, -64.0295) -> (44.0103, -65.7615)
  line L1319 (41.0103, -64.0295) -> (42.0103, -62.2974)
  line L1320 (42.0103, -62.2974) -> (44.0103, -62.2974)
  line L1321 (44.0103, -62.2974) -> (45.0103, -64.0295)
  line L1322 (46.7423, -68.4936) -> (45.7423, -66.7615)
  line L1323 (49.7423, -66.7615) -> (48.7423, -68.4936)
  line L1324 (46.7423, -65.0295) -> (48.7423, -65.0295)
  line L1325 (48.7423, -65.0295) -> (49.7423, -66.7615)
  line L1326 (48.7423, -68.4936) -> (46.7423, -68.4936)
  line L1327 (45.7423, -66.7615) -> (46.7423, -65.0295)
  line L1328 (51.4744, -65.7615) -> (50.4744, -64.0295)
  line L1329 (53.4744, -65.7615) -> (51.4744, -65.7615)
  line L1330 (54.4744, -64.0295) -> (53.4744, -65.7615)
  line L1331 (50.4744, -64.0295) -> (51.4744, -62.2974)
  line L1332 (51.4744, -62.2974) -> (53.4744, -62.2974)
  line L1333 (53.4744, -62.2974) -> (54.4744, -64.0295)
  line L1334 (56.2064, -68.4936) -> (55.2064, -66.7615)
  line L1335 (59.2064, -66.7615) -> (58.2064, -68.4936)
  line L1336 (56.2064, -65.0295) -> (58.2064, -65.0295)
  line L1337 (58.2064, -65.0295) -> (59.2064, -66.7615)
  line L1338 (58.2064, -68.4936) -> (56.2064, -68.4936)
  line L1339 (55.2064, -66.7615) -> (56.2064, -65.0295)
  line L1340 (60.9385, -65.7615) -> (59.9385, -64.0295)
  line L1341 (62.9385, -65.7615) -> (60.9385, -65.7615)
  line L1342 (63.9385, -64.0295) -> (62.9385, -65.7615)
  line L1343 (59.9385, -64.0295) -> (60.9385, -62.2974)
  line L1344 (60.9385, -62.2974) -> (62.9385, -62.2974)
  line L1345 (62.9385, -62.2974) -> (63.9385, -64.0295)
  line L1346 (65.6705, -68.4936) -> (64.6705, -66.7615)
  line L1347 (68.6705, -66.7615) -> (67.6705, -68.4936)
  line L1348 (65.6705, -65.0295) -> (67.6705, -65.0295)
  line L1349 (67.6705, -65.0295) -> (68.6705, -66.7615)
  line L1350 (67.6705, -68.4936) -> (65.6705, -68.4936)
  line L1351 (64.6705, -66.7615) -> (65.6705, -65.0295)
  line L1352 (70.4026, -65.7615) -> (69.4026, -64.0295)
  line L1353 (72.4026, -65.7615) -> (70.4026, -65.7615)
  line L1354 (73.4026, -64.0295) -> (72.4026, -65.7615)
  line L1355 (69.4026, -64.0295) -> (70.4026, -62.2974)
  line L1356 (70.4026, -62.2974) -> (72.4026, -62.2974)
  line L1357 (72.4026, -62.2974) -> (73.4026, -64.0295)
  line L1358 (75.1346, -68.4936) -> (74.1346, -66.7615)
  line L1359 (78.1346, -66.7615) -> (77.1346, -68.4936)
  line L1360 (75.1346, -65.0295) -> (77.1346, -65.0295)
  line L1361 (77.1346, -65.0295) -> (78.1346, -66.7615)
  line L1362 (77.1346, -68.4936) -> (75.1346, -68.4936)
  line L1363 (74.1346, -66.7615) -> (75.1346, -65.0295)
  line L1364 (79.8667, -65.7615) -> (78.8667, -64.0295)
  line L1365 (81.8667, -65.7615) -> (79.8667, -65.7615)
  line L1366 (82.8667, -64.0295) -> (81.8667, -65.7615)
  line L1367 (78.8667, -64.0295) -> (79.8667, -62.2974)
  line L1368 (79.8667, -62.2974) -> (81.8667, -62.2974)
  line L1369 (81.8667, -62.2974) -> (82.8667, -64.0295)
  line L1370 (18.35, -73.9577) -> (17.35, -72.2256)
  line L1371 (21.35, -72.2256) -> (20.35, -73.9577)
  line L1372 (18.35, -70.4936) -> (20.35, -70.4936)
  line L1373 (20.35, -70.4936) -> (21.35, -72.2256)
  line L1374 (20.35, -73.9577) -> (18.35, -73.9577)
  line L1375 (17.35, -72.2256) -> (18.35, -70.4936)
  line L1376 (23.0821, -71.2256) -> (22.0821, -69.4936)
  line L1377 (25.0821, -71.2256) -> (23.0821, -71.2256)
  line L1378 (26.0821, -69.4936) -> (25.0821, -71.2256)
  line L1379 (22.0821, -69.4936) -> (23.0821, -67.7615)
  line L1380 (23.0821, -67.7615) -> (25.0821, -67.7615)
  line L1381 (25.0821, -67.7615) -> (26.0821, -69.4936)
  line L1382 (27.8141, -73.9577) -> (26.8141, -72.2256)
  line L1383 (30.8141, -72.2256) -> (29.8141, -73.9577)
  line L1384 (27.8141, -70.4936) -> (29.8141, -70.4936)
  line L1385 (29.8141, -70.4936) -> (30.8141, -72.2256)
  line L1386 (29.8141, -73.9577) -> (27.8141, -73.9577)
  line L1387 (26.8141, -72.2256) -> (27.8141, -70.4936)
  line L1388 (32.5462, -71.2256) -> (31.5462, -69.4936)
  line L1389 (34.5462, -71.2256) -> (32.5462, -71.2256)
  line L1390 (35.5462, -69.4936) -> (34.5462, -71.2256)
  line L1391 (31.5462, -69.4936) -> (32.5462, -67.7615)
  line L1392 (32.5462, -67.7615) -> (34.5462, -67.7615)
  line L1393 (34.5462, -67.7615) -> (35.5462, -69.4936)
  line L1394 (37.2782, -73.9577) -> (36.2782, -72.2256)
  line L1395 (40.2782, -72.2256) -> (39.2782, -73.9577)
  line L1396 (37.2782, -70.4936) -> (39.2782, -70.4936)
  line L1397 (39.2782, -70.4936) -> (40.2782, -72.2256)
  line L1398 (39.2782, -73.9577) -> (37.2782, -73.9577)
  line L1399 (36.2782, -72.2256) -> (37.2782, -70.4936)
  line L1400 (42.0103, -71.2256) -> (41.0103, -69.4936)
  line L1401 (44.0103, -71.2256) -> (42.0103, -71.2256)
  line L1402 (45.0103, -69.4936) -> (44.0103, -71.2256)
  line L1403 (41.0103, -69.4936) -> (42.0103, -67.7615)
  line L1404 (42.0103, -67.7615) -> (44.0103, -67.7615)
  line L1405 (44.0103, -67.7615) -> (45.0103, -69.4936)
  line L1406 (46.7423, -73.9577) -> (45.7423, -72.2256)
  line L1407 (49.7423, -72.2256) -> (48.7423, -73.9577)
  line L1408 (46.7423, -70.4936) -> (48.7423, -70.4936)
  line L1409 (48.7423, -70.4936) -> (49.7423, -72.2256)
  line L1410 (48.7423, -73.9577) -> (46.7423, -73.9577)
  line L1411 (45.7423, -72.2256) -> (46.7423, -70.4936)
  line L1412 (51.4744, -71.2256) -> (50.4744, -69.4936)
  line L1413 (53.4744, -71.2256) -> (51.4744, -71.2256)
  line L1414 (54.4744, -69.4936) -> (53.4744, -71.2256)
  line L1415 (50.4744, -69.4936) -> (51.4744, -67.7615)
  line L1416 (51.4744, -67.7615) -> (53.4744, -67.7615)
  line L1417 (53.4744, -67.7615) -> (54.4744, -69.4936)
  line L1418 (56.2064, -73.9577) -> (55.2064, -72.2256)
  line L1419 (59.2064, -72.2256) -> (58.2064, -73.9577)
  line L1420 (56.2064, -70.4936) -> (58.2064, -70.4936)
  line L1421 (58.2064, -70.4936) -> (59.2064, -72.2256)
  line L1422 (58.2064, -73.9577) -> (56.2064, -73.9577)
  line L1423 (55.2064, -72.2256) -> (56.2064, -70.4936)
  line L1424 (60.9385, -71.2256) -> (59.9385, -69.4936)
  line L1425 (62.9385, -71.2256) -> (60.9385, -71.2256)
  line L1426 (63.9385, -69.4936) -> (62.9385, -71.2256)
  line L1427 (59.9385, -69.4936) -> (60.9385, -67.7615)
  line L1428 (60.9385, -67.7615) -> (62.9385, -67.7615)
  line L1429 (62.9385, -67.7615) -> (63.9385, -69.4936)
  line L1430 (65.6705, -73.9577) -> (64.6705, -72.2256)
  line L1431 (68.6705, -72.2256) -> (67.6705, -73.9577)
  line L1432 (65.6705, -70.4936) -> (67.6705, -70.4936)
  line L1433 (67.6705, -70.4936) -> (68.6705, -72.2256)
  line L1434 (67.6705, -73.9577) -> (65.6705, -73.9577)
  line L1435 (64.6705, -72.2256) -> (65.6705, -70.4936)
  line L1436 (70.4026, -71.2256) -> (69.4026, -69.4936)
  line L1437 (72.4026, -71.2256) -> (70.4026, -71.2256)
  line L1438 (73.4026, -69.4936) -> (72.4026, -71.2256)
  line L1439 (69.4026, -69.4936) -> (70.4026, -67.7615)
  line L1440 (70.4026, -67.7615) -> (72.4026, -67.7615)
  line L1441 (72.4026, -67.7615) -> (73.4026, -69.4936)
  line L1442 (75.1346, -73.9577) -> (74.1346, -72.2256)
  line L1443 (78.1346, -72.2256) -> (77.1346, -73.9577)
  line L1444 (75.1346, -70.4936) -> (77.1346, -70.4936)
  line L1445 (77.1346, -70.4936) -> (78.1346, -72.2256)
  line L1446 (77.1346, -73.9577) -> (75.1346, -73.9577)
  line L1447 (74.1346, -72.2256) -> (75.1346, -70.4936)
  line L1448 (79.8667, -71.2256) -> (78.8667, -69.4936)
  line L1449 (81.8667, -71.2256) -> (79.8667, -71.2256)
  line L1450 (82.8667, -69.4936) -> (81.8667, -71.2256)
  line L1451 (78.8667, -69.4936) -> (79.8667, -67.7615)
  line L1452 (79.8667, -67.7615) -> (81.8667, -67.7615)
  line L1453 (81.8667, -67.7615) -> (82.8667, -69.4936)
  line L1454 (18.35, -79.4218) -> (17.35, -77.6897)
  line L1455 (21.35, -77.6897) -> (20.35, -79.4218)
  line L1456 (18.35, -75.9577) -> (20.35, -75.9577)
  line L1457 (20.35, -75.9577) -> (21.35, -77.6897)
  line L1458 (20.35, -79.4218) -> (18.35, -79.4218)
  line L1459 (17.35, -77.6897) -> (18.35, -75.9577)
  line L1460 (23.0821, -76.6897) -> (22.0821, -74.9577)
  line L1461 (25.0821, -76.6897) -> (23.0821, -76.6897)
  line L1462 (26.0821, -74.9577) -> (25.0821, -76.6897)
  line L1463 (22.0821, -74.9577) -> (23.0821, -73.2256)
  line L1464 (23.0821, -73.2256) -> (25.0821, -73.2256)
  line L1465 (25.0821, -73.2256) -> (26.0821, -74.9577)
  line L1466 (27.8141, -79.4218) -> (26.8141, -77.6897)
  line L1467 (30.8141, -77.6897) -> (29.8141, -79.4218)
  line L1468 (27.8141, -75.9577) -> (29.8141, -75.9577)
  line L1469 (29.8141, -75.9577) -> (30.8141, -77.6897)
  line L1470 (29.8141, -79.4218) -> (27.8141, -79.4218)
  line L1471 (26.8141, -77.6897) -> (27.8141, -75.9577)
  line L1472 (32.5462, -76.6897) -> (31.5462, -74.9577)
  line L1473 (34.5462, -76.6897) -> (32.5462, -76.6897)
  line L1474 (35.5462, -74.9577) -> (34.5462, -76.6897)
  line L1475 (31.5462, -74.9577) -> (32.5462, -73.2256)
  line L1476 (32.5462, -73.2256) -> (34.5462, -73.2256)
  line L1477 (34.5462, -73.2256) -> (35.5462, -74.9577)
  line L1478 (37.2782, -79.4218) -> (36.2782, -77.6897)
  line L1479 (40.2782, -77.6897) -> (39.2782, -79.4218)
  line L1480 (37.2782, -75.9577) -> (39.2782, -75.9577)
  line L1481 (39.2782, -75.9577) -> (40.2782, -77.6897)
  line L1482 (39.2782, -79.4218) -> (37.2782, -79.4218)
  line L1483 (36.2782, -77.6897) -> (37.2782, -75.9577)
  line L1484 (42.0103, -76.6897) -> (41.0103, -74.9577)
  line L1485 (44.0103, -76.6897) -> (42.0103, -76.6897)
  line L1486 (45.0103, -74.9577) -> (44.0103, -76.6897)
  line L1487 (41.0103, -74.9577) -> (42.0103, -73.2256)
  line L1488 (42.0103, -73.2256) -> (44.0103, -73.2256)
  line L1489 (44.0103, -73.2256) -> (45.0103, -74.9577)
  line L1490 (46.7423, -79.4218) -> (45.7423, -77.6897)
  line L1491 (49.7423, -77.6897) -> (48.7423, -79.4218)
  line L1492 (46.7423, -75.9577) -> (48.7423, -75.9577)
  line L1493 (48.7423, -75.9577) -> (49.7423, -77.6897)
  line L1494 (48.7423, -79.4218) -> (46.7423, -79.4218)
  line L1495 (45.7423, -77.6897) -> (46.7423, -75.9577)
  line L1496 (51.4744, -76.6897) -> (50.4744, -74.9577)
  line L1497 (53.4744, -76.6897) -> (51.4744, -76.6897)
  line L1498 (54.4744, -74.9577) -> (53.4744, -76.6897)
  line L1499 (50.4744, -74.9577) -> (51.4744, -73.2256)
  line L1500 (51.4744, -73.2256) -> (53.4744, -73.2256)
  line L1501 (53.4744, -73.2256) -> (54.4744, -74.9577)
  line L1502 (56.2064, -79.4218) -> (55.2064, -77.6897)
  line L1503 (59.2064, -77.6897) -> (58.2064, -79.4218)
  line L1504 (56.2064, -75.9577) -> (58.2064, -75.9577)
  line L1505 (58.2064, -75.9577) -> (59.2064, -77.6897)
  line L1506 (58.2064, -79.4218) -> (56.2064, -79.4218)
  line L1507 (55.2064, -77.6897) -> (56.2064, -75.9577)
  line L1508 (60.9385, -76.6897) -> (59.9385, -74.9577)
  line L1509 (62.9385, -76.6897) -> (60.9385, -76.6897)
  line L1510 (63.9385, -74.9577) -> (62.9385, -76.6897)
  line L1511 (59.9385, -74.9577) -> (60.9385, -73.2256)
  line L1512 (60.9385, -73.2256) -> (62.9385, -73.2256)
  line L1513 (62.9385, -73.2256) -> (63.9385, -74.9577)
  line L1514 (65.6705, -79.4218) -> (64.6705, -77.6897)
  line L1515 (68.6705, -77.6897) -> (67.6705, -79.4218)
  line L1516 (65.6705, -75.9577) -> (67.6705, -75.9577)
  line L1517 (67.6705, -75.9577) -> (68.6705, -77.6897)
  line L1518 (67.6705, -79.4218) -> (65.6705, -79.4218)
  line L1519 (64.6705, -77.6897) -> (65.6705, -75.9577)
  line L1520 (70.4026, -76.6897) -> (69.4026, -74.9577)
  line L1521 (72.4026, -76.6897) -> (70.4026, -76.6897)
  line L1522 (73.4026, -74.9577) -> (72.4026, -76.6897)
  line L1523 (69.4026, -74.9577) -> (70.4026, -73.2256)
  line L1524 (70.4026, -73.2256) -> (72.4026, -73.2256)
  line L1525 (72.4026, -73.2256) -> (73.4026, -74.9577)
  line L1526 (75.1346, -79.4218) -> (74.1346, -77.6897)
  line L1527 (78.1346, -77.6897) -> (77.1346, -79.4218)
  line L1528 (75.1346, -75.9577) -> (77.1346, -75.9577)
  line L1529 (77.1346, -75.9577) -> (78.1346, -77.6897)
  line L1530 (77.1346, -79.4218) -> (75.1346, -79.4218)
  line L1531 (74.1346, -77.6897) -> (75.1346, -75.9577)
  line L1532 (79.8667, -76.6897) -> (78.8667, -74.9577)
  line L1533 (81.8667, -76.6897) -> (79.8667, -76.6897)
  line L1534 (82.8667, -74.9577) -> (81.8667, -76.6897)
  line L1535 (78.8667, -74.9577) -> (79.8667, -73.2256)
  line L1536 (79.8667, -73.2256) -> (81.8667, -73.2256)
  line L1537 (81.8667, -73.2256) -> (82.8667, -74.9577)
  point P0 (0, 0)
  point P1 (19.35, 15.2)
  point P2 (24.0821, 17.9321)
  point P3 (28.8141, 15.2)
  point P4 (24.0821, 12.4679)
  point P5 (19.35, 9.7359)
  point P6 (28.8141, 15.2)
  point P7 (33.5462, 17.9321)
  point P8 (38.2782, 15.2)
  point P9 (43.0103, 17.9321)
  point P10 (47.7423, 15.2)
  point P11 (52.4744, 17.9321)
  point P12 (57.2064, 15.2)
  point P13 (61.9385, 17.9321)
  point P14 (66.6705, 15.2)
  point P15 (71.4026, 17.9321)
  point P16 (76.1346, 15.2)
  point P17 (80.8667, 17.9321)
  point P18 (19.35, 9.7359)
  point P19 (24.0821, 12.4679)
  point P20 (28.8141, 9.7359)
  point P21 (33.5462, 12.4679)
  point P22 (38.2782, 9.7359)
  point P23 (43.0103, 12.4679)
  point P24 (47.7423, 9.7359)
  point P25 (52.4744, 12.4679)
  point P26 (57.2064, 9.7359)
  point P27 (61.9385, 12.4679)
  point P28 (66.6705, 9.7359)
  point P29 (71.4026, 12.4679)
  point P30 (76.1346, 9.7359)
  point P31 (80.8667, 12.4679)
  point P32 (19.35, 4.2718)
  point P33 (24.0821, 7.0038)
  point P34 (28.8141, 4.2718)
  point P35 (33.5462, 7.0038)
  point P36 (38.2782, 4.2718)
  point P37 (43.0103, 7.0038)
  point P38 (47.7423, 4.2718)
  point P39 (52.4744, 7.0038)
  point P40 (57.2064, 4.2718)
  point P41 (61.9385, 7.0038)
  point P42 (66.6705, 4.2718)
  point P43 (71.4026, 7.0038)
  point P44 (76.1346, 4.2718)
  point P45 (80.8667, 7.0038)
  point P46 (19.35, -1.1923)
  point P47 (24.0821, 1.5397)
  point P48 (28.8141, -1.1923)
  point P49 (33.5462, 1.5397)
  point P50 (38.2782, -1.1923)
  point P51 (43.0103, 1.5397)
  point P52 (47.7423, -1.1923)
  point P53 (52.4744, 1.5397)
  point P54 (57.2064, -1.1923)
  point P55 (61.9385, 1.5397)
  point P56 (66.6705, -1.1923)
  point P57 (71.4026, 1.5397)
  point P58 (76.1346, -1.1923)
  point P59 (80.8667, 1.5397)
  point P60 (19.35, -6.6564)
  point P61 (24.0821, -3.9244)
  point P62 (28.8141, -6.6564)
  point P63 (33.5462, -3.9244)
  point P64 (38.2782, -6.6564)
  point P65 (43.0103, -3.9244)
  point P66 (47.7423, -6.6564)
  point P67 (52.4744, -3.9244)
  point P68 (57.2064, -6.6564)
  point P69 (61.9385, -3.9244)
  point P70 (66.6705, -6.6564)
  point P71 (71.4026, -3.9244)
  point P72 (76.1346, -6.6564)
  point P73 (80.8667, -3.9244)
  point P74 (19.35, -12.1205)
  point P75 (24.0821, -9.3885)
  point P76 (28.8141, -12.1205)
  point P77 (33.5462, -9.3885)
  point P78 (38.2782, -12.1205)
  point P79 (43.0103, -9.3885)
  point P80 (47.7423, -12.1205)
  point P81 (52.4744, -9.3885)
  point P82 (57.2064, -12.1205)
  point P83 (61.9385, -9.3885)
  point P84 (66.6705, -12.1205)
  point P85 (71.4026, -9.3885)
  point P86 (76.1346, -12.1205)
  point P87 (80.8667, -9.3885)
  point P88 (19.35, -17.5846)
  point P89 (24.0821, -14.8526)
  point P90 (28.8141, -17.5846)
  point P91 (33.5462, -14.8526)
  point P92 (38.2782, -17.5846)
  point P93 (43.0103, -14.8526)
  point P94 (47.7423, -17.5846)
  point P95 (52.4744, -14.8526)
  point P96 (57.2064, -17.5846)
  point P97 (61.9385, -14.8526)
  point P98 (66.6705, -17.5846)
  point P99 (71.4026, -14.8526)
  point P100 (76.1346, -17.5846)
  point P101 (80.8667, -14.8526)
  point P102 (19.35, -23.0487)
  point P103 (24.0821, -20.3167)
  point P104 (28.8141, -23.0487)
  point P105 (33.5462, -20.3167)
  point P106 (38.2782, -23.0487)
  point P107 (43.0103, -20.3167)
  point P108 (47.7423, -23.0487)
  point P109 (52.4744, -20.3167)
  point P110 (57.2064, -23.0487)
  point P111 (61.9385, -20.3167)
  point P112 (66.6705, -23.0487)
  point P113 (71.4026, -20.3167)
  point P114 (76.1346, -23.0487)
  point P115 (80.8667, -20.3167)
  point P116 (19.35, -28.5128)
  point P117 (24.0821, -25.7808)
  point P118 (28.8141, -28.5128)
  point P119 (33.5462, -25.7808)
  point P120 (38.2782, -28.5128)
  point P121 (43.0103, -25.7808)
  point P122 (47.7423, -28.5128)
  point P123 (52.4744, -25.7808)
  point P124 (57.2064, -28.5128)
  point P125 (61.9385, -25.7808)
  point P126 (66.6705, -28.5128)
  point P127 (71.4026, -25.7808)
  point P128 (76.1346, -28.5128)
  point P129 (80.8667, -25.7808)
  point P130 (19.35, -33.9769)
  point P131 (24.0821, -31.2449)
  point P132 (28.8141, -33.9769)
  point P133 (33.5462, -31.2449)
  point P134 (38.2782, -33.9769)
  point P135 (43.0103, -31.2449)
  point P136 (47.7423, -33.9769)
  point P137 (52.4744, -31.2449)
  point P138 (57.2064, -33.9769)
  point P139 (61.9385, -31.2449)
  point P140 (66.6705, -33.9769)
  point P141 (71.4026, -31.2449)
  point P142 (76.1346, -33.9769)
  point P143 (80.8667, -31.2449)
  point P144 (19.35, -39.441)
  point P145 (24.0821, -36.709)
  point P146 (28.8141, -39.441)
  point P147 (33.5462, -36.709)
  point P148 (38.2782, -39.441)
  point P149 (43.0103, -36.709)
  point P150 (47.7423, -39.441)
  point P151 (52.4744, -36.709)
  point P152 (57.2064, -39.441)
  point P153 (61.9385, -36.709)
  point P154 (66.6705, -39.441)
  point P155 (71.4026, -36.709)
  point P156 (76.1346, -39.441)
  point P157 (80.8667, -36.709)
  point P158 (19.35, -44.9051)
  point P159 (24.0821, -42.1731)
  point P160 (28.8141, -44.9051)
  point P161 (33.5462, -42.1731)
  point P162 (38.2782, -44.9051)
  point P163 (43.0103, -42.1731)
  point P164 (47.7423, -44.9051)
  point P165 (52.4744, -42.1731)
  point P166 (57.2064, -44.9051)
  point P167 (61.9385, -42.1731)
  point P168 (66.6705, -44.9051)
  point P169 (71.4026, -42.1731)
  point P170 (76.1346, -44.9051)
  point P171 (80.8667, -42.1731)
  point P172 (19.35, -50.3692)
  point P173 (24.0821, -47.6372)
  point P174 (28.8141, -50.3692)
  point P175 (33.5462, -47.6372)
  point P176 (38.2782, -50.3692)
  point P177 (43.0103, -47.6372)
  point P178 (47.7423, -50.3692)
  point P179 (52.4744, -47.6372)
  point P180 (57.2064, -50.3692)
  point P181 (61.9385, -47.6372)
  point P182 (66.6705, -50.3692)
  point P183 (71.4026, -47.6372)
  point P184 (76.1346, -50.3692)
  point P185 (80.8667, -47.6372)
  point P186 (19.35, -55.8333)
  point P187 (24.0821, -53.1013)
  point P188 (28.8141, -55.8333)
  point P189 (33.5462, -53.1013)
  point P190 (38.2782, -55.8333)
  point P191 (43.0103, -53.1013)
  point P192 (47.7423, -55.8333)
  point P193 (52.4744, -53.1013)
  point P194 (57.2064, -55.8333)
  point P195 (61.9385, -53.1013)
  point P196 (66.6705, -55.8333)
  point P197 (71.4026, -53.1013)
  point P198 (76.1346, -55.8333)
  point P199 (80.8667, -53.1013)
  dimension "d38" = 2
  dimension "d40" = 5
  dimension "d41" = 2.5
  dimension "d42" = 2.5
  dimension "d43" = 2
  dimension "d44" = 2
  dimension "d45" = 2
  dimension "d46" = 2
  dimension "d47" = 9.4641
  dimension "d48" = 2
  dimension "d49" = 2
  dimension "d50" = 2
  dimension "d51" = 2
  dimension "d52" = 2
  dimension "d53" = 2
  dimension "d54" = 5.4641
  dimension "d57" = 9.4641
  dimension "d60" = 5.4641
  constraints: 3066 end point, 6 horizontal, 2 perpendicular, 1 collinear, 1 vertical, 3314 other
  measures "d38" distance of L8.end L4.start
  measures "d40" distance between parallel lines of L10 L1
  measures "d41" distance from line of point (19.35, 15.2) L1
  measures "d42" distance from line of point (19.35, 15.2) L0
  measures "d43" distance of L15.end L11.start
  measures "d44" distance of L21.end L17.start
  measures "d45" distance between parallel lines of L14 L4
  measures "d46" distance between parallel lines of L12 L21
  measures "d47" distance of L20.end L7.end
  measures "d48" distance of L30.start L25.start
  measures "d49" distance of L36.start L31.start
  measures "d50" distance between parallel lines of L5 L29
  measures "d51" distance between parallel lines of L6 L36
  measures "d52" distance between parallel lines of L28 L31
  measures "d53" distance between parallel lines of L13 L30
  measures "d54" distance between parallel lines of L36 L9
  measures "d57" distance of L6.end L38.start
  measures "d60" distance of L6.end L110.start
extrude "Extrusion4" add sketch "Sketch7" against normal blind 2 contours L0 L1 L29 L28 L27 L26 L25 L131 L128 L129 L130 L133 L143 L140 L141 L142 L145 L155 L152 L153 L154 L157 L167 L164 L165 L166 L169 L179 L176 L177 L178 L181 L2 L3 L1529 L1528 L1531 L1517 L1516 L1519 L1505 L1504 L1507 L1493 L1492 L1495 L1481 L1480 L1483 L1469 L1468 L1471 | L1471 L1468 L1469 L3 | L3 L1469 L1467 L1470 L1466 L1471 | L1 L25 L26 L27 L28 L29 | L1483 L1480 L1481 L3 | L1 L133 L130 L129 L128 L131 | L1495 L1492 L1493 L3 | L1 L145 L142 L141 L140 L143 | L1507 L1504 L1505 L3 | L1 L157 L154 L153 L152 L155 | L1519 L1516 L1517 L3 | L1 L169 L166 L165 L164 L167 | L1531 L1528 L1529 L3 | L1 L181 L178 L177 L176 L179